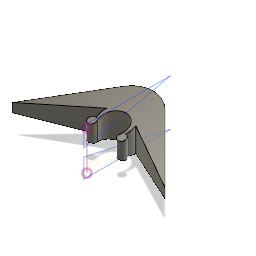
rampClipv1 (Autodesk Fusion 360 design; units mm, degrees)
part number: rampClip
Autodesk Fusion 360 part; units mm, degrees
note: some values were not read from the file. Set by a fixed rule: which sketch regions a step uses.
sketch "main body" plane through (0, 0, 0) normal (0, 1, 0) x (1, 0, 0) in component "main"
  arc A0 (-7.5849, 2.5435) -> (7.6843, 2.225) centre (0, 0) ccw
  line L0 (-7.5849, 2.5435) -> (-38.6454, -15.3377)
  line L1 (-38.6454, -15.3377) -> (-0.1069, 25.2491)
  line L2 (-0.1069, 25.2491) -> (39.4777, -14.3181)
  line L3 (39.4777, -14.3181) -> (7.6843, 2.225)
  dimension "d1" = 8
  measures "d1" radius of A0
extrude "Extrude1" add sketch "main body" along normal blind 20 in component "main"
fillet "Fillet1" radius 15 1 edges at (-0.1069, 10, -25.2491) in component "main"
sketch "main hole" plane through (0, 20, 0) normal (0, 1, 0) x (-1, 0, 0) in component "main"
  arc A0 (-10.7778, -14.3691) -> (10.704, -14.0888) centre (-0.1736, -3.7602) ccw
  line L0 (10.704, -14.0888) -> (38.6454, 15.3377)
  line L1 (38.6454, 15.3377) -> (7.5849, -2.5435)
  line L2 (-7.6843, -2.225) -> (-39.4777, 14.3181)
  line L3 (-39.4777, 14.3181) -> (-10.7778, -14.3691)
  circle A1 centre (-0.0035, 1.6197) radius 6.5
  line L4 (-10.0035, 3.8921) -> (9.9387, 3.8921)
  line L5 (9.9387, 3.8921) -> (9.9387, 20.1413)
  line L6 (9.9387, 20.1413) -> (-10.0035, 20.1413)
  line L7 (-10.0035, 20.1413) -> (-10.0035, 3.8921)
  line L8 (-10.0035, 3.8921) -> (9.9387, 20.1413) construction
  line L9 (9.9387, 3.8921) -> (-10.0035, 20.1413) construction
  dimension "d5" = 13
  measures "d5" diameter of A1
extrude "Extrude5" cut sketch "main hole" against normal blind 20 in component "main"
extrude "Extrude3" cut sketch "main hole" against normal blind 20 contours A1 L4 | A1 L4 in component "main"
sketch "rounded borders" plane through (0, 0, 0) normal (0, 1, 0) x (1, 0, 0) in component "main"
  circle A0 centre (-7.8046, -4.9719) radius 2
  circle A1 centre (7.7907, -4.9961) radius 2
  dimension "d16" = 4
  dimension "d17" = 4
  measures "d16" diameter of A0
  measures "d17" diameter of A1
extrude "Extrude6" add sketch "rounded borders" along normal blind 20 in component "main"
sketch "cut sides" plane through (0, 0, 0) normal (1, 0, 0) x (0, 0, -1) in component "main"
  line L0 (28, 22) -> (-17, 12)
  line L1 (-15.3377, 0) -> (-15.3377, 20)
  line L2 (-17, 12) -> (-17, 22)
  line L3 (-17, 22) -> (28, 22)
  line L4 (28, -2) -> (-17, 8)
  line L5 (-17, 8) -> (-17, -2)
  line L6 (-17, -2) -> (28, -2)
extrude "Extrude7" cut sketch "cut sides" along normal mid plane 100 in component "main"
sketch "Sketch9" plane through (0, 0, 0) normal (1, 0, 0) x (0, 1, 0) in component "main"
  circle A0 centre (10, -18.5) radius 0.825
  dimension "d22" = 1.65
  measures "d22" diameter of A0
extrude "Extrude8" cut sketch "Sketch9" along normal mid plane 40 in component "main"
component "main" placed x (1, 0, 0) y (0, 1, 0) z (0, 0, 1) at (0, 0, 0)
